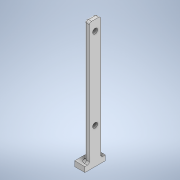
# Autodesk Inventor part: baseB
Saved by Autodesk Inventor 2021.4 (Build 254397000, 397)
## iProperties
Created: 2023-11-06
Part Number: baseB
Material: 一般
Document SubType Name: Modeling
Designer: ryusei
Density: 1 g/cm^3
Appearance: 既定
Author: ryusei
Autodesk Inventor part; units mm, degrees
ref_plane "YZ Plane" through (0, 0, 0) normal (1, 0, 0) x (0, 1, 0)
ref_plane "XZ Plane" through (0, 0, 0) normal (0, 1, 0) x (-1, 0, 0)
ref_plane "XY Plane" through (0, 0, 0) normal (0, 0, 1) x (1, 0, 0)
sketch "スケッチ1" plane through (0, 0, 0) normal (0, 1, 0) x (-1, 0, 0)
  line L0 (5, -10) -> (-5, -10)
  line L1 (-5, -10) -> (-5, 10)
  line L2 (-5, 10) -> (5, 10)
  line L3 (5, 10) -> (5, -10)
  line L4 (5, -10) -> (-5, 10) construction
  line L5 (-5, -10) -> (5, 10) construction
  point P0 (0, 0)
  dimension "d0" = 10
  dimension "d1" = 20
  constraints: 12 end point, 2 midpoint, 2 parallel, 1 horizontal, 1 perpendicular
  measures "d0" distance of L1.end L2.end
  measures "d1" distance of L0.end L1.end
extrude "押し出し1" add sketch "スケッチ1" along normal blind 5
sketch "スケッチ4" plane through (0, 5, 0) normal (0, 1, 0) x (1, 0, 0)
  line L0 (5, 5.5) -> (0, 5.5)
  line L1 (0, 5.5) -> (0, -5.5)
  line L2 (0, -5.5) -> (5, -5.5)
  line L3 (5, -5.5) -> (5, 5.5)
  line L4 (5, -10) -> (5, 10) projected
  point P0 (0, 0)
  dimension "d11" = 5
  dimension "d12" = 11
  dimension "d13" = 5
  dimension "d14" = 5.5
  constraints: 8 end point, 2 parallel, 1 horizontal, 1 perpendicular
  measures "d11" distance of L2.end L1.end
  measures "d12" distance of L1.end L0.end
  measures "d13" distance between parallel lines of L4 L1
  measures "d14" distance from line of point (0, 0) L0
extrude "押し出し4" add sketch "スケッチ4" along normal blind 120
sketch "スケッチ6" plane through (5, 0, 10) normal (1, 0, 0) x (0, 0, -1)
  line L0 (4.5, 5) -> (15.5, 5) projected
  line L1 (15.5, 5) -> (15.5, 125) projected
  point P0 (10, 0)
  point P1 (10, 35)
  point P2 (10, 115)
  dimension "d30" = 30
  dimension "d31" = 80
  dimension "d32" = 5.5
  dimension "d33" = 5.5
  measures "d30" distance from line of L0 point (10, 35)
  measures "d31" distance of point (10, 115) point (10, 35)
  measures "d32" distance from line of L1 point (10, 115)
  measures "d33" distance from line of L1 point (10, 35)
hole "穴2" at (5, 35, 0) at (5, 115, 0) direction (-1, 0, 0) diameter 4.9 end through all
fillet "フィレット3" radius 2 8 edges at (2.5, 125, 5.5) (2.5, 125, -5.5) (0, 125, 0) (0, 65, 5.5) (0, 65, -5.5) (2.5, 5, 5.5) (0, 5, 0) (2.5, 5, -5.5)
